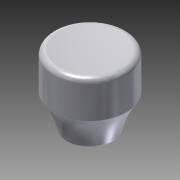
# Autodesk Inventor part: pushbutton
Saved by Autodesk Inventor 2013 (Build 170138000, 138)
## iProperties
Created: 2013-01-11
Part Number: pushbutton
Material: Generic
Document SubType Name: Modeling
Designer: md
Density: 1 g/cm^3
Author: md
Autodesk Inventor part; units mm, degrees
ref_plane "YZ Plane" through (0, 0, 0) normal (1, 0, 0) x (0, 1, 0)
ref_plane "XZ Plane" through (0, 0, 0) normal (0, 1, 0) x (-1, 0, 0)
ref_plane "XY Plane" through (0, 0, 0) normal (0, 0, 1) x (1, 0, 0)
sketch "Sketch1" plane through (0, 0, 0) normal (0, 1, 0) x (-1, 0, 0)
  line L0 (1.7668, 0) -> (1.7668, 7)
  line L1 (1.7668, 7) -> (0.0668, 7)
  line L2 (0.0668, 7) -> (0.0668, 14)
  line L3 (4.7168, 0) -> (1.7668, 0)
  arc A0 (0.0668, 14) -> (7.5, 14.7071) centre (0.3407, 50.5458) ccw
  arc A1 (7.5, 7) -> (4.7168, 0) centre (20.9678, -2.4081) ccw
  line L4 (1.7668, 7) -> (7.5, 7) construction
  line L5 (7.5, 7) -> (7.5, 0) construction
  line L6 (7.5, 7) -> (7.5, 14.7071)
  point P0 (0, 0)
  dimension "d0" = 1.7
  dimension "d5" = 7
  dimension "d10" = 0
  dimension "d11" = 36.5468
  dimension "d12" = 7
  dimension "d16" = 14.7071
  dimension "d17" = 16.4285
  dimension "d18" = 2.95
  dimension "d20" = 20.9678
  dimension "d21" = 5.7332
  dimension "d22" = 7
  constraints: 14 end point, 4 point on circle, 3 parallel, 2 centre point, 2 perpendicular, 1 collinear, 1 vertical
  measures "d0" distance of L0.end L1.end
  measures "d5" distance of L0.start L0.end
  measures "d10" distance from line of point (0, 0) L3
  measures "d11" radius of A0
  measures "d12" distance of L1.end L2.end
  measures "d16" distance from line of L6.end L3
  measures "d17" radius of A1
  measures "d18" distance of L3.start L0.start
  measures "d20" horizontal distance of A1.centre point (0, 0)
  measures "d21" distance between parallel lines of L5 L0
  measures "d22" distance from line of L5.end L1
revolve "Revolution1" add sketch "Sketch1" angle 360 about axis through (-0.0668, 0, 7) along (0, 0, 1)
fillet "Fillet1" radius 1 2 edges at (4.5832, 0, 0) (7.3664, 0, 14.7071)
equation "\"d0\" = 0.5 * LSH_Durchmesser + epsilon"
equation "\"d15\" = Rundung"
equation "\"LSH_Durchmesser\" = 3.2"
equation "\"epsilon\" = 0.1"
equation "\"Taster_Durchmesser\" = 15"
equation "\"Rundung\" = 1"
body "Solid1"
